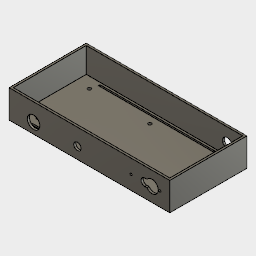
charlesBox_middle (Autodesk Fusion 360 design; units mm, degrees)
Autodesk Fusion 360 part; units mm, degrees
note: some values were not read from the file. Set by a fixed rule: which sketch regions a step uses.
sketch "Sketch1" plane through (0, 0, 0) normal (0, 1, 0) x (1, 0, 0)
  line L0 (75, 35) -> (-75, 35)
  line L1 (-75, 35) -> (-75, -35)
  line L2 (-75, -35) -> (75, -35)
  line L3 (75, -35) -> (75, 35)
  line L4 (75, 35) -> (-75, -35) construction
  line L5 (-75, 35) -> (75, -35) construction
  dimension "d1" = 150
  dimension "d2" = 70
  measures "d1" distance of L0.start L0.end
  measures "d2" distance of L0.start L2.end
extrude "Extrude1" add sketch "Sketch1" along normal blind 3
sketch "Sketch2" plane through (0, 0, 0) normal (0, 1, 0) x (1, 0, 0)
  line L0 (-75, 35) -> (-75, -35)
  line L1 (75, 35) -> (-75, 35)
  line L2 (75, -35) -> (75, 35)
  line L3 (-75, -35) -> (75, -35)
  line L4 (77, 37) -> (-77, 37)
  line L5 (-77, 37) -> (-77, -37)
  line L6 (-77, -37) -> (77, -37)
  line L7 (77, -37) -> (77, 37)
  line L8 (77, 37) -> (-77, -37) construction
  line L9 (-77, 37) -> (77, -37) construction
  dimension "d5" = 2
  dimension "d6" = 2
  measures "d5" distance of L1 L4
  measures "d6" distance of L0 L5
extrude "Extrude2" add sketch "Sketch2" along normal blind 27
sketch "Sketch3" plane through (0, 0, 0) normal (0, 1, 0) x (1, 0, 0)
  line L0 (-60, 31.5) -> (60, 31.5)
  line L1 (60, 31.5) -> (60, 33)
  line L2 (60, 33) -> (-60, 33)
  line L3 (-60, 33) -> (-60, 31.5)
  line L4 (-60.5, -31.5) -> (60.5, -31.5)
  line L5 (60.5, -31.5) -> (60.5, -33)
  line L6 (60.5, -33) -> (-60.5, -33)
  line L7 (-60.5, -33) -> (-60.5, -31.5)
  line L8 (0, 31.5) -> (0, -31.5)
  dimension "d9" = 63
  dimension "d10" = 1.5
  dimension "d11" = 120
  measures "d9" distance of L8.start L8.end
  measures "d10" distance of L4.start L6.end
  measures "d11" distance of L0.start L0.end
extrude "Extrude3" cut sketch "Sketch3" along normal through all
sketch "Sketch4" plane through (0, 0, 0) normal (0, 1, 0) x (1, 0, 0)
  line L0 (23, 29) -> (-65, 29) construction
  line L1 (-65, 29) -> (-65, -29) construction
  line L2 (-65, -29) -> (23, -29) construction
  line L3 (23, -29) -> (23, 29) construction
  line L4 (23, 29) -> (-65, -29) construction
  line L5 (-65, 29) -> (23, -29) construction
  circle A0 centre (-61.5, 24.5) radius 1.55
  circle A1 centre (-61.5, -24.5) radius 1.55
  circle A2 centre (-3.5, -24.5) radius 1.55
  circle A3 centre (-3.5, 24.5) radius 1.55
  line L6 (-61.5, 24.5) -> (-61.5, -24.5) construction
  line L7 (-75, -35) -> (-75, 35)
  point P0 (-21, 0)
  point P1 (-61.5, 0)
  dimension "d13" = 58
  dimension "d14" = 88
  dimension "d15" = 3.1
  dimension "d16" = 58
  dimension "d17" = 49
  dimension "d18" = 3.5
  dimension "d19" = 10
  measures "d13" distance of L0.end L1.end
  measures "d14" distance of L0.start L0.end
  measures "d15" diameter of A0
  measures "d16" distance of A0.centre A3.centre
  measures "d17" distance of A0.centre A1.centre
  measures "d18" distance of L1 A0.centre
  measures "d19" distance of L1 L7
extrude "Extrude4" cut sketch "Sketch4" along normal through all
sketch "Sketch5" plane through (0, 0, 0) normal (0, 0, 1) x (1, 0, 0)
  circle A0 centre (60, 13.5) radius 4.5
  line L0 (64.2, 15.1155) -> (64.2, 11.8845)
  line L1 (55.8, 15.1155) -> (55.8, 11.8845)
  dimension "d21" = 9
  dimension "d22" = 60
  dimension "d23" = 13.5
  dimension "d25" = 8.4
  measures "d21" diameter of A0
  measures "d22" distance of origin A0.centre
  measures "d23" distance of origin A0.centre
  measures "d25" distance of L0 L1
extrude "Extrude5" cut sketch "Sketch5" against normal through all contours A0 L0 L1
sketch "Sketch6" plane through (0, 0, 0) normal (0, 0, 1) x (1, 0, 0)
  circle A0 centre (39.9, 13.5) radius 1
  circle A1 centre (67.5, 13.5) radius 1
  line L0 (53, 17) -> (55.1266, 17)
  line L1 (53, 10) -> (55.1266, 10)
  arc A2 (55.1266, 10) -> (55.1266, 17) centre (60, 13.5) ccw
  arc A3 (53, 17) -> (53, 10) centre (53, 13.5) ccw
  dimension "d26" = 13.5
  dimension "d27" = 2
  dimension "d28" = 27.6
  dimension "d29" = 12
  dimension "d30" = 7.5
  dimension "d31" = 60
  dimension "d33" = 7
  dimension "d34" = 7
  measures "d26" distance of origin A0.centre
  measures "d27" diameter of A0
  measures "d28" distance of A0.centre A1.centre
  measures "d29" diameter of A2
  measures "d30" distance of A1.centre A2.centre
  measures "d31" distance of origin A2.centre
  measures "d33" diameter of A3
  measures "d34" distance of A2.centre A3.centre
extrude "Extrude6" cut sketch "Sketch6" along normal through all
sketch "Sketch7" plane through (0, 0, 0) normal (0, 0, 1) x (1, 0, 0)
  circle A0 centre (-53.5, 10) radius 6
  circle A1 centre (-11.5, 11) radius 3.5
  dimension "d35" = 12
  dimension "d36" = 10
  dimension "d37" = 53.5
  dimension "d39" = 7
  dimension "d40" = 1
  dimension "d41" = 42
  measures "d35" diameter of A0
  measures "d36" distance of origin A0.centre
  measures "d37" distance of origin A0.centre
  measures "d39" diameter of A1
  measures "d40" distance of A0.centre A1.centre
  measures "d41" distance of A0.centre A1.centre
extrude "Extrude7" cut sketch "Sketch7" along normal blind 37
equation "d6 = d5"
equation "d23 = ( 27 / 2 ) * 1 mm"
equation "d26 = ( 27 / 2 ) * 1 mm"
equation "d37 = 61.5 mm - 8 mm"
